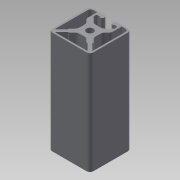
# Autodesk Inventor part: 40-4001
Saved by Autodesk Inventor 2013 (Build 170138000, 138)
## iProperties
Created: 2014-04-23
Part Number: 40-4001
Material: Generic
Document SubType Name: Modeling
Designer: Ross Bowman
Density: 1 g/cm^3
Engineer: Ross Bowman
Catalog Web Link: 8020.net
Vendor: 80/20 Inc.
Company: 80/20 Inc.
Author: Ross Bowman
Keywords: 80/20 , 8020 , T-Slot , Extrusion
Material: 6105-T5 Aluminum
Autodesk Inventor part; units mm, degrees
ref_plane "YZ Plane" through (0, 0, 0) normal (1, 0, 0) x (0, 1, 0)
ref_plane "XZ Plane" through (0, 0, 0) normal (0, 1, 0) x (-1, 0, 0)
ref_plane "XY Plane" through (0, 0, 0) normal (0, 0, 1) x (1, 0, 0)
sketch "Sketch1" plane through (0, 0, 0) normal (0, 0, 1) x (1, 0, 0)
  circle A0 centre (0, 0) radius 3.4
  arc A1 (15.4108, -18.35) -> (15.5882, -17.9217) centre (15.4108, -18.0991) ccw
  line L0 (-15.4108, -18.35) -> (15.4108, -18.35)
  arc A2 (-15.5882, -17.9217) -> (-15.4108, -18.35) centre (-15.4108, -18.0991) ccw
  line L1 (-9.7291, -12.0626) -> (-15.5882, -17.9217)
  arc A3 (-9.1903, -11.8394) -> (-9.7291, -12.0626) centre (-9.1903, -12.6014) ccw
  line L2 (-8.7439, -11.8394) -> (-9.1903, -11.8394)
  arc A4 (-8.7439, -11.8394) -> (-8.2051, -11.6162) centre (-8.7439, -11.0774) ccw
  line L3 (-5.6651, -9.0762) -> (-8.2051, -11.6162)
  arc A5 (-2.3065, -7.685) -> (-5.6651, -9.0762) centre (-2.3065, -12.4348) ccw
  line L4 (2.3065, -7.685) -> (-2.3065, -7.685)
  arc A6 (5.6651, -9.0762) -> (2.3065, -7.685) centre (2.3065, -12.4348) ccw
  line L5 (8.2051, -11.6162) -> (5.6651, -9.0762)
  arc A7 (8.2051, -11.6162) -> (8.7439, -11.8394) centre (8.7439, -11.0774) ccw
  line L6 (9.1903, -11.8394) -> (8.7439, -11.8394)
  arc A8 (9.7291, -12.0626) -> (9.1903, -11.8394) centre (9.1903, -12.6014) ccw
  line L7 (15.5882, -17.9217) -> (9.7291, -12.0626)
  arc A9 (11.7694, -8.6739) -> (11.5462, -8.1351) centre (11.0074, -8.6739) ccw
  line L8 (9.0762, -5.6651) -> (11.5462, -8.1351)
  arc A10 (7.685, -2.3065) -> (9.0762, -5.6651) centre (12.4348, -2.3065) ccw
  line L9 (7.685, 2.3065) -> (7.685, -2.3065)
  arc A11 (9.0762, 5.6651) -> (7.685, 2.3065) centre (12.4348, 2.3065) ccw
  line L10 (11.0322, 7.6211) -> (9.0762, 5.6651)
  arc A12 (11.0322, 7.6211) -> (11.9621, 9.8662) centre (8.7871, 9.8662) ccw
  line L11 (11.9621, 18.5086) -> (11.9621, 9.8662)
  arc A13 (12.3431, 18.8896) -> (11.9621, 18.5086) centre (12.3431, 18.5086) ccw
  line L12 (15.556, 18.8896) -> (12.3431, 18.8896)
  arc A14 (18.35, 16.0956) -> (15.556, 18.8896) centre (15.556, 16.0956) ccw
  line L13 (18.35, -15.3747) -> (18.35, 16.0956)
  arc A15 (17.8962, -15.5627) -> (18.35, -15.3747) centre (18.0841, -15.3747) ccw
  line L14 (11.9926, -9.6591) -> (17.8962, -15.5627)
  arc A16 (11.7694, -9.1203) -> (11.9926, -9.6591) centre (12.5314, -9.1203) ccw
  line L15 (11.7694, -8.6739) -> (11.7694, -9.1203)
  arc A17 (-9.0762, -5.6651) -> (-7.685, -2.3065) centre (-12.4348, -2.3065) ccw
  line L16 (-11.5462, -8.1351) -> (-9.0762, -5.6651)
  arc A18 (-11.5462, -8.1351) -> (-11.7694, -8.6739) centre (-11.0074, -8.6739) ccw
  line L17 (-11.7694, -9.1203) -> (-11.7694, -8.6739)
  arc A19 (-11.9926, -9.6591) -> (-11.7694, -9.1203) centre (-12.5314, -9.1203) ccw
  line L18 (-17.8962, -15.5627) -> (-11.9926, -9.6591)
  arc A20 (-18.35, -15.3747) -> (-17.8962, -15.5627) centre (-18.0841, -15.3747) ccw
  line L19 (-18.35, 16.0956) -> (-18.35, -15.3747)
  arc A21 (-15.556, 18.8896) -> (-18.35, 16.0956) centre (-15.556, 16.0956) ccw
  line L20 (-12.3431, 18.8896) -> (-15.556, 18.8896)
  arc A22 (-11.9621, 18.5086) -> (-12.3431, 18.8896) centre (-12.3431, 18.5086) ccw
  line L21 (-11.9621, 9.8662) -> (-11.9621, 18.5086)
  arc A23 (-11.9621, 9.8662) -> (-11.0322, 7.6211) centre (-8.7871, 9.8662) ccw
  line L22 (-9.0762, 5.6651) -> (-11.0322, 7.6211)
  arc A24 (-7.685, 2.3065) -> (-9.0762, 5.6651) centre (-12.4348, 2.3065) ccw
  line L23 (-7.685, -2.3065) -> (-7.685, 2.3065)
  arc A25 (20, 16.825) -> (16.825, 20) centre (16.825, 16.825) ccw
  line L24 (16.825, 20) -> (5.6287, 20)
  arc A26 (5.6287, 20) -> (4.06, 18.2867) centre (5.6287, 18.4252) ccw
  line L25 (4.06, 18.2867) -> (4.06, 17.5148)
  arc A27 (4.06, 17.5148) -> (5.6348, 15.94) centre (5.6348, 17.5148) ccw
  line L26 (5.6348, 15.94) -> (6.8724, 15.94)
  line L27 (6.8724, 15.94) -> (6.899, 16.702)
  line L28 (6.899, 16.702) -> (9.015, 16.702)
  arc A28 (10.285, 15.432) -> (9.015, 16.702) centre (9.015, 15.432) ccw
  line L29 (10.285, 15.432) -> (10.285, 14.0643)
  arc A29 (10.0246, 13.4357) -> (10.285, 14.0643) centre (9.396, 14.0643) ccw
  line L30 (10.0246, 13.4357) -> (5.6651, 9.0762)
  arc A30 (2.3065, 7.685) -> (5.6651, 9.0762) centre (2.3065, 12.4348) ccw
  line L31 (2.3065, 7.685) -> (-2.3065, 7.685)
  arc A31 (-5.6651, 9.0762) -> (-2.3065, 7.685) centre (-2.3065, 12.4348) ccw
  line L32 (-5.6651, 9.0762) -> (-10.0246, 13.4357)
  arc A32 (-10.285, 14.0643) -> (-10.0246, 13.4357) centre (-9.396, 14.0643) ccw
  line L33 (-10.285, 14.0643) -> (-10.285, 15.432)
  arc A33 (-9.015, 16.702) -> (-10.285, 15.432) centre (-9.015, 15.432) ccw
  line L34 (-9.015, 16.702) -> (-6.899, 16.702)
  line L35 (-6.899, 16.702) -> (-6.8724, 15.94)
  line L36 (-6.8724, 15.94) -> (-5.6348, 15.94)
  arc A34 (-5.6348, 15.94) -> (-4.06, 17.5148) centre (-5.6348, 17.5148) ccw
  line L37 (-4.06, 17.5148) -> (-4.06, 18.2867)
  arc A35 (-4.06, 18.2867) -> (-5.6287, 20) centre (-5.6287, 18.4252) ccw
  line L38 (-5.6287, 20) -> (-16.825, 20)
  arc A36 (-16.825, 20) -> (-20, 16.825) centre (-16.825, 16.825) ccw
  line L39 (-20, 16.825) -> (-20, -16.825)
  arc A37 (-20, -16.825) -> (-16.825, -20) centre (-16.825, -16.825) ccw
  line L40 (-16.825, -20) -> (16.825, -20)
  arc A38 (16.825, -20) -> (20, -16.825) centre (16.825, -16.825) ccw
  line L41 (20, -16.825) -> (20, 16.825)
  constraints: 84 end point, 76 point on circle, 39 centre point
extrude "Extrusion1" add sketch "Sketch1" against normal blind 100
body "Solid1"
